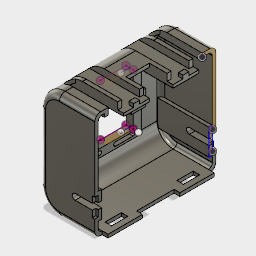
body_rear (Autodesk Fusion 360 design; units mm, degrees)
Autodesk Fusion 360 part; units mm, degrees
sketch "スケッチ1" plane through (0, 0, 0) normal (0, 1, 0) x (1, 0, 0)
  line L0 (0, 0) -> (28, 0)
  line L1 (28, 0) -> (28, -30.8)
  line L2 (28, -30.8) -> (0, -30.8)
  line L3 (0, -30.8) -> (0, 0)
  line L4 (28, 0) -> (28, -3.75)
  line L5 (28, -3.75) -> (31, -3.75)
  line L6 (31, -3.75) -> (31, -21.285)
  line L7 (31, -21.285) -> (28, -21.285)
  line L8 (28, -21.285) -> (28, -3.75)
  line L9 (28, -3.75) -> (28, -8.37)
  line L10 (28, -8.37) -> (28.15, -8.37)
  line L11 (28.15, -8.37) -> (24.85, -8.37)
  line L12 (24.85, -8.37) -> (24.85, -16.67)
  line L13 (24.85, -16.67) -> (28.15, -16.67)
  line L14 (28.15, -16.67) -> (28.15, -8.37)
  dimension "d1" = 28
  dimension "d2" = 30.8
  dimension "d12" = 3.75
  dimension "d13" = 3
  dimension "d14" = 17.535
  dimension "d15" = 4.62
  dimension "d16" = 0.15
  dimension "d17" = 3.3
  dimension "d18" = 8.3
  constraint horizontal L0
  constraint vertical L1
  constraint horizontal L2
  constraint vertical L3
  constraint horizontal L5
  constraint vertical L6
  constraint horizontal L7
  constraint vertical L8
  constraint horizontal L11
  constraint vertical L12
  constraint horizontal L13
  constraint vertical L14
sketch "スケッチ2" plane through (0, 0, 0) normal (0, 0, 1) x (1, 0, 0)
  line L0 (0, 0) -> (28, 0)
  line L1 (28, 0) -> (28, 54.6)
  line L2 (28, 54.6) -> (0, 54.6)
  line L3 (0, 54.6) -> (0, 0)
  line L4 (28, 0) -> (28, 12.1)
  line L5 (28, 12.1) -> (18, 12.1)
  line L6 (18, 12.1) -> (18, 15.1)
  line L7 (18, 15.1) -> (28, 15.1)
  line L8 (28, 15.1) -> (28, 12.1)
  line L9 (28, 12.1) -> (26.788, 12.1)
  line L10 (26.788, 12.1) -> (26.788, 8.781)
  line L11 (26.788, 8.781) -> (28, 8.781)
  line L12 (28, 8.781) -> (28, 12.1)
  line L13 (28, 15.1) -> (26.788, 15.1)
  line L14 (26.788, 15.1) -> (26.788, 18.419)
  line L15 (26.788, 18.419) -> (28, 18.419)
  line L16 (28, 18.419) -> (28, 15.1)
  circle A0 centre (18, 13.6) radius 1.5
  dimension "d3" = 28
  dimension "d4" = 54.6
  dimension "d5" = 12.1
  dimension "d6" = 10
  dimension "d7" = 3
  dimension "d8" = 1.212
  dimension "d9" = 3.319
  dimension "d10" = 3.319
  dimension "d11" = 1.212
  constraint horizontal L0
  constraint vertical L1
  constraint horizontal L2
  constraint vertical L3
  constraint horizontal L5
  constraint vertical L6
  constraint horizontal L7
  constraint vertical L8
  constraint horizontal L9
  constraint vertical L10
  constraint horizontal L11
  constraint vertical L12
  constraint midpoint L9
  constraint midpoint L11
  constraint horizontal L13
  constraint vertical L14
  constraint horizontal L15
  constraint vertical L16
  constraint coincident A0
  constraint tangent L5 A0
sketch "スケッチ3" plane through (0, 0, 0) normal (1, 0, 0) x (0, 0, -1)
  line L0 (0, 0) -> (-30.8, 0)
  line L1 (-30.8, 0) -> (-30.8, 54.6)
  line L2 (-30.8, 54.6) -> (0, 54.6)
  line L3 (0, 54.6) -> (0, 0)
  line L4 (-30.8, 0) -> (0, 0)
  line L5 (-30.8, 54.6) -> (-30.8, 40.48)
  line L6 (-30.8, 40.48) -> (-17.72, 40.48)
  line L7 (-17.72, 40.48) -> (-17.72, 14.32)
  line L8 (-17.72, 14.32) -> (-30.8, 14.32)
  line L9 (-30.8, 14.32) -> (-30.8, 40.48)
  line L10 (-17.72, 14.32) -> (-17.72, 40.48)
  line L11 (-17.72, 40.48) -> (-17.72, 27.4)
  line L12 (-17.72, 27.4) -> (-17.72, 31.4)
  line L13 (-17.72, 27.4) -> (-17.72, 23.4)
  line L14 (-17.72, 23.4) -> (-20.87, 23.4)
  line L15 (-20.87, 23.4) -> (-20.87, 31.4)
  line L16 (-20.87, 31.4) -> (-17.72, 31.4)
  line L17 (-17.72, 31.4) -> (-17.72, 23.4)
  line L18 (-17.72, 23.4) -> (-13.6, 23.4)
  line L19 (-13.6, 23.4) -> (-13.6, 31.4)
  line L20 (-13.6, 31.4) -> (-17.72, 31.4)
  line L21 (-17.72, 31.4) -> (-17.72, 23.4)
  line L22 (-30.8, 14.32) -> (-30.8, 10.2)
  line L23 (-30.8, 40.48) -> (-30.8, 44.6)
  line L24 (-30.8, 10.2) -> (-30.8, 44.6)
  line L25 (-30.8, 44.6) -> (-13.6, 44.6)
  line L26 (-13.6, 44.6) -> (-13.6, 10.2)
  line L27 (-13.6, 10.2) -> (-30.8, 10.2)
  line L28 (-17.72, 14.32) -> (-17.72, 13.32) construction
  line L29 (-17.72, 13.32) -> (-26.72, 13.32)
  line L30 (-26.72, 13.32) -> (-26.72, 11.32)
  line L31 (-26.72, 11.32) -> (-17.72, 11.32)
  line L32 (-17.72, 11.32) -> (-17.72, 13.32)
  circle A0 centre (-17.72, 12.32) radius 1
  circle A1 centre (-26.72, 12.32) radius 1
  line L33 (-17.72, 40.48) -> (-17.72, 41.48) construction
  line L34 (-17.72, 41.48) -> (-26.72, 41.48)
  line L35 (-26.72, 41.48) -> (-26.72, 43.48)
  line L36 (-26.72, 43.48) -> (-17.72, 43.48)
  line L37 (-17.72, 43.48) -> (-17.72, 41.48)
  circle A2 centre (-17.72, 42.48) radius 1
  circle A3 centre (-26.72, 42.48) radius 1
  dimension "d23" = 14.12
  dimension "d24" = 13.08
  dimension "d25" = 26.16
  dimension "d26" = 4
  dimension "d27" = 4
  dimension "d28" = 3.15
  dimension "d29" = 8
  dimension "d30" = 4.12
  dimension "d31" = 4.12
  dimension "d32" = 4.12
  dimension "d45" = 1
  dimension "d46" = 9
  dimension "d47" = 2
  dimension "d48" = 1
  dimension "d49" = 2
  dimension "d50" = 9
  constraint perpendicular L0 L1
  constraint parallel L0 L2
  constraint parallel L1 L3
  constraint parallel L0 L4
  constraint horizontal L6
  constraint vertical L7
  constraint horizontal L8
  constraint vertical L9
  constraint midpoint L10
  constraint horizontal L14
  constraint vertical L15
  constraint horizontal L16
  constraint vertical L17
  constraint horizontal L18
  constraint vertical L19
  constraint horizontal L20
  constraint perpendicular L24 L25
  constraint parallel L24 L26
  constraint parallel L25 L27
  constraint parallel L23 L24
  constraint horizontal L29
  constraint vertical L30
  constraint horizontal L31
  constraint vertical L32
  constraint midpoint L32
  constraint coincident A0
  constraint tangent L31 A0
  constraint midpoint L30
  constraint coincident A1
  constraint tangent L29 A1
  constraint horizontal L34
  constraint vertical L35
  constraint horizontal L36
  constraint vertical L37
  constraint midpoint L37
  constraint coincident A2
  constraint tangent L34 A2
  constraint midpoint L35
  constraint coincident A3
  constraint tangent L34 A3
extrude "押し出し3" add sketch "スケッチ1" along normal blind 1.75 contours L0 L1 L2 L3 L4 L8 L9 L11 L12 L13 | L1 L5 L6 L7 L8 L9 L10 L11 L13 L14 makes body 1
extrude "押し出し4" add sketch "スケッチ2" along normal blind 1.75 contours L0 L1 L2 L3 L4 L5 L7 L10 L11 L14 L15 A0 bodies 1
extrude "押し出し5" add sketch "スケッチ3" along normal blind 5.9 separate body contours L7 L10 L11 L12 L13 L17 L18 L19 L20 L21 L26 | L7 L10 L11 L12 L13 L14 L15 L16 L17 L21 makes body 2
extrude "押し出し6" add sketch "スケッチ3" along normal blind 3.7 contours L1 L7 L8 L10 L18 L22 L24 L26 L27 | L1 L5 L6 L7 L10 L11 L20 L23 L24 L25 L26 bodies 2
extrude "押し出し7" add sketch "スケッチ3" along normal blind 1.75 contours L0 L1 L2 L3 L4 L5 L19 L25 L26 L27 bodies 1 2
extrude "押し出し8" cut sketch "スケッチ3" along normal blind 3.7 contours L7 L10 L11 L12 L13 L14 L15 L16 L17 L21 bodies 1
ref_plane "作業平面1" through (14, 54.6, 15.4) normal (0, 1, 0) x (-1, 0, 0)
sketch "スケッチ4" plane through (14, 54.6, 15.4) normal (0, 1, 0) x (1, 0, 0)
  line L0 (-14, 15.4) -> (14, 15.4)
  line L1 (14, 15.4) -> (14, -15.4)
  line L2 (14, -15.4) -> (-14, -15.4)
  line L3 (-14, -15.4) -> (-14, 15.4)
  line L4 (14, -15.4) -> (8, -15.4)
  line L5 (8, -15.4) -> (8, -9.4)
  line L6 (8, -9.4) -> (14, -9.4)
  line L7 (14, -9.4) -> (14, -15.4)
  line L8 (14, -9.4) -> (14, -7.4)
  line L9 (14, -7.4) -> (14, 1.71)
  line L10 (14, 1.71) -> (14, 3.71)
  line L11 (14, 3.71) -> (14, 8.5)
  line L12 (14, -9.4) -> (14, 3.71)
  line L13 (14, 3.71) -> (17, 3.71)
  line L14 (17, 3.71) -> (17, -9.4)
  line L15 (17, -9.4) -> (14, -9.4)
  line L16 (17, -2.845) -> (17, -1.32)
  line L17 (17, -2.845) -> (17, -4.37)
  line L18 (17, -4.37) -> (17, -1.32)
  line L19 (17, -1.32) -> (14.7, -1.32)
  line L20 (14.7, -1.32) -> (14.7, -4.37)
  line L21 (14.7, -4.37) -> (17, -4.37)
  line L22 (14, 1.71) -> (14, -7.4)
  line L23 (14, -7.4) -> (-14, -7.4)
  line L24 (-14, -7.4) -> (-14, 1.71)
  line L25 (-14, 1.71) -> (14, 1.71)
  line L26 (17, 3.71) -> (17, -9.4)
  line L27 (17, -9.4) -> (-14, -9.4)
  line L28 (-14, -9.4) -> (-14, 3.71)
  line L29 (-14, 3.71) -> (17, 3.71)
  line L30 (14, 8.5) -> (14, 3.71)
  line L31 (14, 3.71) -> (-7.5, 3.71)
  line L32 (-7.5, 3.71) -> (-7.5, 8.5)
  line L33 (-7.5, 8.5) -> (14, 8.5)
  circle A0 centre (-7.5, 6.105) radius 2.395
  line L34 (14, 8.5) -> (14, 10.5)
  line L35 (14, 10.5) -> (14, 8.5)
  line L36 (14, 8.5) -> (-14, 8.5)
  line L37 (-14, 8.5) -> (-14, 10.5)
  line L38 (-14, 10.5) -> (14, 10.5)
  line L39 (-14, -15.4) -> (-14, 15.4)
  dimension "d58" = 6
  dimension "d59" = 6
  dimension "d60" = 2
  dimension "d61" = 9.11
  dimension "d62" = 2
  dimension "d63" = 4.79
  dimension "d64" = 3
  dimension "d66" = 1.525
  dimension "d67" = 1.525
  dimension "d68" = 21.5
  dimension "d69" = 2
  constraint horizontal L0
  constraint vertical L1
  constraint horizontal L2
  constraint vertical L3
  constraint horizontal L4
  constraint vertical L5
  constraint horizontal L6
  constraint vertical L7
  constraint perpendicular L12 L13
  constraint parallel L12 L14
  constraint parallel L13 L15
  constraint perpendicular L6 L12
  constraint midpoint L14
  constraint perpendicular L18 L19
  constraint parallel L18 L20
  constraint parallel L19 L21
  constraint parallel L16 L18
  constraint perpendicular L22 L23
  constraint parallel L22 L24
  constraint parallel L23 L25
  constraint parallel L12 L22
  constraint perpendicular L26 L27
  constraint parallel L26 L28
  constraint parallel L27 L29
  constraint perpendicular L30 L31
  constraint parallel L30 L32
  constraint parallel L31 L33
  constraint perpendicular L29 L30
  constraint midpoint L32
  constraint coincident A0
  constraint perpendicular L35 L36
  constraint parallel L35 L37
  constraint parallel L36 L38
  constraint perpendicular L33 L35
extrude "押し出し9" add sketch "スケッチ4" against normal blind 1.75 contours L0 L1 L3 L38 L39 | L1 L3 L33 L34 L35 L36 L37 L38 L39 | L3 L29 A0 L36 L39 | L1 L3 L10 L12 L25 L28 L29 L31 L39 | L1 L8 L9 L10 L12 L13 L14 L15 L19 L20 L21 L22 L26 L27 L29 | L1 L3 L9 L12 L22 L23 L24 L25 L28 L39 | L1 L3 L6 L8 L12 L23 L27 L28 L39 | L14 L16 L17 L18 L19 L20 L21 L26 | L2 L3 L5 L27 L39 bodies 1
fillet "フィレット1" radius 8.25 2 edges at (1.75, 52.85, 16.275) (1.75, 1.75, 16.275) on bodies 1
fillet "フィレット2" radius 2 5 edges at (19, 52.85, 1.75) (4.1664, 50.4336, 1.75) (1.75, 27.3, 1.75) (4.1664, 4.1664, 1.75) (19, 1.75, 1.75) on bodies 1
fillet "フィレット3" radius 10 2 edges at (0, 0, 15.4) (0, 54.6, 15.4) on bodies 1
fillet "フィレット4" radius 3 5 edges at (19, 54.6, 0) (2.9289, 51.6711, 0) (0, 27.3, 0) (2.9289, 2.9289, 0) (19, 0, 0) on bodies 1
sketch "スケッチ5" plane through (31, 0, 0) normal (1, 0, 0) x (0, 0, -1)
  line L0 (-11.69, 54.6) -> (-24.8, 54.6)
  line L1 (-24.8, 54.6) -> (-24.8, 52.85)
  line L2 (-24.8, 52.85) -> (-11.69, 52.85)
  line L3 (-11.69, 52.85) -> (-11.69, 54.6)
  line L4 (-24.8, 52.85) -> (-11.69, 52.85)
  line L5 (-11.69, 52.85) -> (-11.69, 49.6)
  line L6 (-11.69, 49.6) -> (-24.8, 49.6)
  line L7 (-24.8, 49.6) -> (-24.8, 52.85)
  dimension "d76" = 3.25
  constraint perpendicular L4 L5
  constraint parallel L4 L6
  constraint parallel L5 L7
sketch "スケッチ6" plane through (28, 0, 0) normal (1, 0, 0) x (0, 0, -1)
  arc A0 (0, 51.6) -> (-3, 54.6) centre (-3, 51.6) ccw
  line L0 (-3, 54.6) -> (-6.9, 54.6)
  line L1 (-6.9, 54.6) -> (-6.9, 52.85)
  line L2 (-6.9, 52.85) -> (-3.75, 52.85)
  arc A1 (-1.75, 50.85) -> (-3.75, 52.85) centre (-3.75, 50.85) ccw
  line L3 (-1.75, 50.85) -> (-1.75, 18.419)
  line L4 (-1.75, 18.419) -> (0, 18.419)
  line L5 (0, 18.419) -> (0, 51.6)
  line L6 (-6.9, 52.85) -> (-4.9, 52.85)
  line L7 (-6.9, 52.85) -> (-4.9, 52.85)
  line L8 (-4.9, 52.85) -> (-4.9, 51.1)
  line L9 (-4.9, 51.1) -> (-6.9, 51.1)
  line L10 (-6.9, 51.1) -> (-6.9, 52.85)
  line L11 (-1.75, 18.419) -> (-1.75, 20.2)
  line L12 (-1.75, 8.781) -> (-1.75, 7)
  line L13 (-1.75, 7) -> (-1.75, 20.2)
  line L14 (-1.75, 20.2) -> (-3.5, 20.2)
  line L15 (-3.5, 20.2) -> (-3.5, 7)
  line L16 (-3.5, 7) -> (-1.75, 7)
  dimension "d77" = 2
  dimension "d78" = 1.75
  dimension "d79" = 1.781
  dimension "d80" = 1.781
  dimension "d81" = 1.75
  constraint perpendicular L7 L8
  constraint parallel L7 L9
  constraint parallel L8 L10
  constraint parallel L6 L7
  constraint perpendicular L13 L14
  constraint parallel L13 L15
  constraint parallel L14 L16
  constraint parallel L12 L13
extrude "押し出し10" add sketch "スケッチ6" against normal blind 27 contours L3 L11 L12 L13 L14 L15 L16 bodies 1
extrude "押し出し11" cut sketch "スケッチ2" along normal blind 7 contours L1 L5 L7 L8 L9 L13 A0 | L6 A0 | L6 A0 bodies 1
extrude "押し出し12" add sketch "スケッチ6" against normal blind 23 contours L2 L6 L7 L8 L9 L10 bodies 1
extrude "押し出し13" add sketch "スケッチ5" against normal blind 26.5 contours L2 L4 L5 L6 L7 bodies 1
extrude "押し出し14" add 1 faces at (4.5, 49.9831, 16.06) along direction (-1, 0, 0) blind 1.6 on bodies 1 bodies 1
extrude "押し出し15" cut sketch "スケッチ4" against normal blind 3.5 contours L1 L8 L9 L10 L12 L13 L14 L15 L19 L20 L21 L22 L26 L27 L29 | L1 L3 L9 L12 L22 L23 L24 L25 L28 L39 bodies 1
extrude "押し出し17" cut 1 faces at (30.2333, 54.6, 18.7533) along direction (0, -1, 0) blind 1.8 on bodies 1 bodies 1
sketch "スケッチ7" plane through (0, 14.32, 0) normal (0, 1, 0) x (-1, 0, 0)
  line L0 (0, 17.72) -> (0, 30.8)
  line L1 (0, 30.8) -> (-3.7, 30.8)
  line L2 (-3.7, 30.8) -> (-3.7, 17.72)
  line L3 (-3.7, 17.72) -> (0, 17.72)
  line L4 (-3.7, 17.72) -> (-1.85, 17.72)
  line L5 (-1.85, 17.72) -> (-1.85, 22.22)
  line L6 (-1.85, 17.72) -> (-6.35, 17.72) construction
  dimension "d102" = 90
  dimension "d103" = 4.5
  constraint midpoint L3
  constraint horizontal L6
  measures "d102" angle of L5 L6
sketch "スケッチ8" plane through (0, 40.48, 0) normal (0, -1, 0) x (1, 0, 0)
  line L0 (0, 30.8) -> (0, 17.72)
  line L1 (0, 17.72) -> (3.7, 17.72)
  line L2 (3.7, 17.72) -> (3.7, 30.8)
  line L3 (3.7, 30.8) -> (0, 30.8)
  line L4 (0, 17.72) -> (1.85, 17.72)
  line L5 (1.85, 17.72) -> (1.85, 22.22)
  dimension "d104" = 4.5
  constraint midpoint L1
sphere "球プリミティブ1" add diameter 1.6 placed x (1, 0, 0) y (0, 0, 1) z (0, -1, 0) at (1.7837, 40.48, 22.2018) bodies 1
sphere "球プリミティブ2" add diameter 1.6 placed x (-1, 0, 0) y (0, 0, 1) z (0, 1, 0) at (1.85, 14.32, 22.22) bodies 1
ref_plane "作業平面2" through (14, 7.16, 30.8) normal (0, 0, 1) x (1, 0, 0)
mirror "ミラー1" about plane through (14, 7.16, 30.8) normal (0, 0, 1) of bodies 1 makes body 3
combine "結合1" operation add target body 3 tool bodies 1
extrude "押し出し18" cut 1 faces at (22, 54.0167, 28.8) along direction (-1, 0, 0) blind 3 on bodies 3 bodies 3
equation "d66 = ( 3.05 / 2 ) * 1 mm"
equation "d67 = ( 3.05 / 2 ) * 1 mm"
